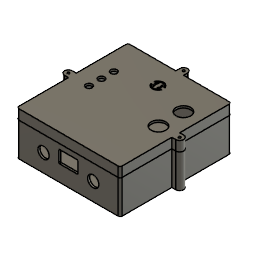
Smart_Chair_Case (Autodesk Fusion 360 design; units mm, degrees)
Autodesk Fusion 360 part; units mm, degrees
note: some values were not read from the file. Set by a fixed rule: which face or edge a step refers to.
sketch "Sketch1" plane through (200, 0, 0) normal (1, 0, 0) x (0, 0, -1)
  line L0 (113.9291, 131.1741) -> (113.9291, 10) construction
  circle A0 centre (113.9291, 70.587) radius 30
  circle A1 centre (113.9291, 70.587) radius 27.5
  circle A2 centre (113.9291, 70.587) radius 25
  circle A3 centre (113.9291, 70.587) radius 22.5
  circle A4 centre (113.9291, 70.587) radius 20
  circle A5 centre (113.9291, 70.587) radius 17.5
  circle A6 centre (113.9291, 70.587) radius 15
  circle A7 centre (113.9291, 70.587) radius 15
  circle A8 centre (113.9291, 70.587) radius 12.5
  circle A9 centre (113.9291, 70.587) radius 10
  circle A10 centre (113.9291, 70.587) radius 7.5
  circle A11 centre (113.9291, 70.587) radius 5
  circle A12 centre (113.9291, 70.587) radius 2.5
  line L1 (71.2868, 76.587) -> (156.5714, 76.587)
  line L2 (156.5714, 76.587) -> (156.5714, 64.587)
  line L3 (156.5714, 64.587) -> (71.2868, 64.587)
  line L4 (71.2868, 64.587) -> (71.2868, 76.587)
  line L5 (71.2868, 76.587) -> (156.5714, 64.587) construction
  line L6 (156.5714, 76.587) -> (71.2868, 64.587) construction
  line L7 (107.9291, 108.7596) -> (119.9291, 108.7596)
  line L8 (119.9291, 108.7596) -> (119.9291, 32.4145)
  line L9 (119.9291, 32.4145) -> (107.9291, 32.4145)
  line L10 (107.9291, 32.4145) -> (107.9291, 108.7596)
  line L11 (107.9291, 108.7596) -> (119.9291, 32.4145) construction
  line L12 (119.9291, 108.7596) -> (107.9291, 32.4145) construction
  line L13 (-90, 0) -> (90, 0)
  line L14 (90, 0) -> (90, 150)
  line L15 (-90, 125) -> (-90, 0)
  line L16 (90, 150) -> (-90, 125)
  point P0 (113.9291, 70.587)
  point P1 (113.9291, 70.587)
  dimension "d204" = 60
  dimension "d205" = 55
  dimension "d206" = 50
  dimension "d207" = 45
  dimension "d208" = 40
  dimension "d209" = 35
  dimension "d210" = 30
  dimension "d211" = 30
  dimension "d212" = 25
  dimension "d213" = 20
  dimension "d214" = 15
  dimension "d215" = 10
  dimension "d216" = 5
  dimension "d217" = 12
  dimension "d218" = 12
  constraint midpoint L0 P1
  constraint concentric A0 A1
  constraint concentric A0 A2
  constraint concentric A2 A3
  constraint concentric A1 A4
  constraint concentric A0 A5
  constraint concentric A1 A6
  constraint concentric A6 A7
  constraint concentric A0 A8
  constraint concentric A7 A9
  constraint concentric A0 A10
  constraint concentric A6 A11
  constraint concentric A3 A12
  constraint horizontal L1
  constraint perpendicular L1 L2
  constraint parallel L1 L3
  constraint parallel L2 L4
  constraint coincident L5 P1
  constraint coincident L6 P1
  constraint coincident P1 P0
  constraint horizontal L7
  constraint perpendicular L7 L8
  constraint parallel L7 L9
  constraint parallel L8 L10
  constraint coincident L11 P1
  constraint coincident L12 P1
  measures "d204" diameter of A0
  measures "d205" diameter of A1
  measures "d206" diameter of A2
  measures "d207" diameter of A3
  measures "d208" diameter of A4
  measures "d209" diameter of A5
  measures "d210" diameter of A6
  measures "d211" diameter of A7
  measures "d212" diameter of A8
  measures "d213" diameter of A9
  measures "d214" diameter of A10
  measures "d215" diameter of A11
  measures "d216" diameter of A12
  measures "d217" distance of L1.end L2.end
  measures "d218" distance of L8.end L9.end
sketch "Sketch1 (2)" plane through (0, 0, 0) normal (0, 1, 0) x (1, 0, 0) in component "Smart_Sprayer_Board_Case"
  line L0 (-77.5, 47.5) -> (77.5, 47.5)
  line L1 (77.5, 47.5) -> (77.5, -47.5)
  line L2 (77.5, -47.5) -> (-77.5, -47.5)
  line L3 (-77.5, -47.5) -> (-77.5, 47.5)
  line L4 (-77.5, 47.5) -> (77.5, -47.5) construction
  line L5 (77.5, 47.5) -> (-77.5, -47.5) construction
  line L6 (-79.25, 49.25) -> (79.25, 49.25)
  line L7 (79.25, 49.25) -> (79.25, -49.25)
  line L8 (79.25, -49.25) -> (-79.25, -49.25)
  line L9 (-79.25, -49.25) -> (-79.25, 49.25)
  line L10 (-79.25, 49.25) -> (79.25, -49.25) construction
  line L11 (79.25, 49.25) -> (-79.25, -49.25) construction
  dimension "d292" = 155
  dimension "d293" = 95
  dimension "d294" = 158.5
  dimension "d295" = 98.5
  constraint horizontal L0
  constraint perpendicular L0 L1
  constraint parallel L0 L2
  constraint parallel L1 L3
  constraint coincident L4 origin
  constraint coincident L5 origin
  constraint horizontal L6
  constraint perpendicular L6 L7
  constraint parallel L6 L8
  constraint parallel L7 L9
  constraint coincident L10 origin
  constraint coincident L11 origin
  measures "d292" distance of L1.end L2.end
  measures "d293" distance of L0.end L1.end
  measures "d294" distance of L7.end L8.end
  measures "d295" distance of L6.end L7.end
extrude "Extrude1" add sketch "Sketch1 (2)" along normal blind 43 makes body 1 in component "Smart_Sprayer_Board_Case"
sketch "Sketch2" plane through (0, 0, 0) normal (0, -1, 0) x (1, 0, 0) in component "Smart_Sprayer_Board_Case"
  line L0 (-77.5, 47.5) -> (77.5, 47.5)
  line L1 (77.5, 47.5) -> (77.5, -47.5)
  line L2 (77.5, -47.5) -> (-77.5, -47.5)
  line L3 (-77.5, -47.5) -> (-77.5, 47.5)
  line L4 (79.25, 49.25) -> (-79.25, 49.25)
  line L5 (-79.25, 49.25) -> (-79.25, -49.25)
  line L6 (-79.25, -49.25) -> (79.25, -49.25)
  line L7 (79.25, -49.25) -> (79.25, 49.25)
extrude "Extrude2" add sketch "Sketch2" along normal blind 1.75 contours L0 L1 L2 L3 | L4 L5 L6 L7 bodies 1 in component "Smart_Sprayer_Board_Case"
sketch "Sketch3" plane through (0, 0, 0) normal (0, 1, 0) x (-1, 0, 0) in component "Smart_Sprayer_Board_Case"
  line L0 (-77.5, 47.5) -> (-77.5, -47.5)
  line L1 (-77.5, -47.5) -> (77.5, -47.5)
  line L2 (77.5, -47.5) -> (77.5, 47.5)
  line L3 (77.5, 47.5) -> (-77.5, 47.5)
  line L4 (70, -41.25) -> (-70, -41.25) construction
  line L5 (-70, -41.25) -> (-70, 41.25) construction
  line L6 (-70, 41.25) -> (70, 41.25) construction
  line L7 (70, 41.25) -> (70, -41.25) construction
  line L8 (70, -41.25) -> (-70, 41.25) construction
  line L9 (-70, -41.25) -> (70, 41.25) construction
  circle A0 centre (70, -41.25) radius 5
  circle A1 centre (-70, -41.25) radius 5
  circle A2 centre (70, 41.25) radius 5
  circle A3 centre (-70, 41.25) radius 5
  dimension "d300" = 140
  dimension "d301" = 82.5
  dimension "d302" = 10
  dimension "d303" = 10
  dimension "d304" = 10
  dimension "d305" = 10
  constraint horizontal L4
  constraint perpendicular L4 L5
  constraint parallel L4 L6
  constraint parallel L5 L7
  constraint coincident L8 origin
  constraint coincident L9 origin
  constraint coincident L4.start L7.end
  constraint coincident L4.end L5.start
  constraint coincident L6.end L7.start
  constraint coincident L5.end L6.start
  measures "d300" distance of L5.end L6.end
  measures "d301" distance of L4.end L5.end
  measures "d302" diameter of A0
  measures "d303" diameter of A1
  measures "d304" diameter of A2
  measures "d305" diameter of A3
extrude "Extrude3" add sketch "Sketch3" along normal blind 3 contours A0 | A1 | A2 | A3 bodies 1 in component "Smart_Sprayer_Board_Case"
sketch "Sketch4" plane through (0, 3, 0) normal (0, 1, 0) x (-1, 0, 0) in component "Smart_Sprayer_Board_Case"
  circle A0 centre (70, -41.25) radius 5
  circle A1 centre (70, -41.25) radius 1
  dimension "d308" = 2
  constraint concentric A0 A1
  measures "d308" diameter of A1
extrude "Extrude4" cut sketch "Sketch4" against normal blind 4 contours A1 bodies 1 in component "Smart_Sprayer_Board_Case"
pattern_linear "R-Pattern1" count 2 spacing 82.5 along (0, 0, 1) count 2 spacing 140 along (1, 0, 0) of "Extrude4" in component "Smart_Sprayer_Board_Case"
sketch "Sketch5" plane through (0, 0, 47.5) normal (0, 0, -1) x (-1, 0, 0) in component "Smart_Sprayer_Board_Case"
  line L0 (-77.5, 0) -> (77.5, 0)
  line L1 (77.5, 0) -> (77.5, 43)
  line L2 (77.5, 43) -> (-77.5, 43)
  line L3 (-77.5, 43) -> (-77.5, 0)
  line L4 (0, 0) -> (0, 18) construction
  line L5 (-8, 25) -> (8, 25)
  line L6 (8, 25) -> (8, 11)
  line L7 (8, 11) -> (-8, 11)
  line L8 (-8, 11) -> (-8, 25)
  line L9 (-8, 25) -> (8, 11) construction
  line L10 (8, 25) -> (-8, 11) construction
  point P0 (0, 18)
  dimension "d315" = 18
  dimension "d316" = 16
  dimension "d317" = 14
  constraint coincident L4.start origin
  constraint perpendicular L0 L4
  constraint horizontal L5
  constraint perpendicular L5 L6
  constraint parallel L5 L7
  constraint parallel L6 L8
  constraint coincident L9 P0
  constraint coincident L10 P0
  constraint coincident P0 L4.end
  measures "d315" distance of L4.start P0
  measures "d316" distance of L6.end L7.end
  measures "d317" distance of L5.end L6.end
extrude "Extrude5" cut sketch "Sketch5" against normal blind 1.75 contours L5 L6 L7 L8 bodies 1 in component "Smart_Sprayer_Board_Case"
sketch "Sketch6" plane through (-79.25, 0, 0) normal (-1, 0, 0) x (0, 0, 1) in component "Smart_Sprayer_Board_Case"
  line L0 (49.25, -1.75) -> (49.25, 43)
  line L1 (49.25, 43) -> (-49.25, 43)
  line L2 (-49.25, 43) -> (-49.25, -1.75)
  line L3 (-49.25, -1.75) -> (49.25, -1.75)
  line L4 (0, 0) -> (0, 25) construction
  line L5 (0, 25) -> (49.25, 25) construction
  line L6 (0, 25) -> (-49.25, 25) construction
  line L7 (0, 25) -> (-21, 25) construction
  line L8 (0, 25) -> (21, 25) construction
  line L9 (-26.5, 30.5) -> (-15.5, 30.5)
  line L10 (-15.5, 30.5) -> (-15.5, 19.5)
  line L11 (-15.5, 19.5) -> (-26.5, 19.5)
  line L12 (-26.5, 19.5) -> (-26.5, 30.5)
  line L13 (-26.5, 30.5) -> (-15.5, 19.5) construction
  line L14 (-15.5, 30.5) -> (-26.5, 19.5) construction
  line L15 (15.5, 30.5) -> (26.5, 30.5)
  line L16 (26.5, 30.5) -> (26.5, 19.5)
  line L17 (26.5, 19.5) -> (15.5, 19.5)
  line L18 (15.5, 19.5) -> (15.5, 30.5)
  line L19 (15.5, 30.5) -> (26.5, 19.5) construction
  line L20 (26.5, 30.5) -> (15.5, 19.5) construction
  point P0 (-21, 25)
  point P1 (21, 25)
  dimension "d320" = 25
  dimension "d321" = 21
  dimension "d322" = 21
  dimension "d323" = 11
  dimension "d324" = 11
  dimension "d325" = 11
  dimension "d326" = 11
  constraint coincident L4.start origin
  constraint perpendicular L3 L4
  constraint coincident L0 L5.end
  constraint perpendicular L0 L5
  constraint coincident L2 L6.end
  constraint perpendicular L2 L6
  constraint perpendicular L4 L7
  constraint perpendicular L4 L8
  constraint horizontal L9
  constraint perpendicular L9 L10
  constraint parallel L9 L11
  constraint parallel L10 L12
  constraint coincident L13 P0
  constraint coincident L14 P0
  constraint coincident P0 L7.end
  constraint horizontal L15
  constraint perpendicular L15 L16
  constraint parallel L15 L17
  constraint parallel L16 L18
  constraint coincident L19 P1
  constraint coincident L20 P1
  constraint coincident P1 L8.end
  measures "d320" distance of L4.start L4.end
  measures "d321" distance of L4.end P0
  measures "d322" distance of L4.end P1
  measures "d323" distance of L10.end L11.end
  measures "d324" distance of L9.end L10.end
  measures "d325" distance of L16.end L17.end
  measures "d326" distance of L15.end L16.end
extrude "Extrude6" cut sketch "Sketch6" against normal blind 1.75 contours L9 L10 L11 L12 | L15 L16 L17 L18 bodies 1 in component "Smart_Sprayer_Board_Case"
sketch "Sketch7" plane through (0, 0, 49.25) normal (0, 0, 1) x (1, 0, 0) in component "Smart_Sprayer_Board_Case"
  line L0 (-8, 11) -> (-8, 25)
  line L1 (-8, 25) -> (8, 25)
  line L2 (8, 25) -> (8, 11)
  line L3 (8, 11) -> (-8, 11)
  line L4 (79.25, -1.75) -> (79.25, 43)
  line L5 (79.25, 43) -> (-79.25, 43)
  line L6 (-79.25, 43) -> (-79.25, -1.75)
  line L7 (-79.25, -1.75) -> (79.25, -1.75)
  line L8 (-8, 18) -> (-79.25, 18) construction
  line L9 (-8, 18) -> (-15, 18) construction
  circle A0 centre (-15, 18) radius 3.5
  dimension "d329" = 7
  dimension "d330" = 7
  constraint midpoint L0 L8.start
  constraint coincident L6 L8.end
  constraint perpendicular L6 L8
  constraint perpendicular L0 L9
  constraint coincident L9.end A0.centre
  measures "d329" distance of L8.start L9.end
  measures "d330" diameter of A0
extrude "Extrude7" cut sketch "Sketch7" against normal blind 1.75 contours A0 bodies 1 in component "Smart_Sprayer_Board_Case"
sketch "Sketch8" plane through (79.25, 0, 0) normal (1, 0, 0) x (0, 0, -1) in component "Smart_Sprayer_Board_Case"
  line L0 (49.25, -1.75) -> (49.25, 43)
  line L1 (49.25, 43) -> (-49.25, 43)
  line L2 (-49.25, 43) -> (-49.25, -1.75)
  line L3 (-49.25, -1.75) -> (49.25, -1.75)
  line L4 (16.5, 29.5) -> (33.5, 29.5)
  line L5 (33.5, 29.5) -> (33.5, 20.5)
  line L6 (33.5, 20.5) -> (16.5, 20.5)
  line L7 (16.5, 20.5) -> (16.5, 29.5)
  line L8 (16.5, 29.5) -> (33.5, 20.5) construction
  line L9 (33.5, 29.5) -> (16.5, 20.5) construction
  point P0 (25, 25)
  dimension "d333" = 17
  dimension "d334" = 9
  constraint horizontal L4
  constraint perpendicular L4 L5
  constraint parallel L4 L6
  constraint parallel L5 L7
  constraint coincident L8 P0
  constraint coincident L9 P0
  measures "d333" distance of L5.end L6.end
  measures "d334" distance of L4.end L5.end
extrude "Extrude8" cut sketch "Sketch8" against normal blind 1.75 contours L4 L5 L6 L7 bodies 1 in component "Smart_Sprayer_Board_Case"
sketch "Sketch9" plane through (0, -1.75, 0) normal (0, -1, 0) x (1, 0, 0) in component "Smart_Sprayer_Board_Case"
  line L0 (79.25, -49.25) -> (79.25, 49.25)
  line L1 (79.25, 49.25) -> (-79.25, 49.25)
  line L2 (-79.25, 49.25) -> (-79.25, -49.25)
  line L3 (-79.25, -49.25) -> (79.25, -49.25)
  line L4 (79.25, -49.25) -> (-79.25, -49.25)
  line L5 (-79.25, -49.25) -> (-79.25, -74.45)
  line L6 (-79.25, -74.45) -> (79.25, -74.45)
  line L7 (79.25, -74.45) -> (79.25, -49.25)
  dimension "d337" = 25.2
  constraint horizontal L4
  constraint vertical L5
  constraint horizontal L6
  constraint vertical L7
  constraint coincident L0.start L3.end
  measures "d337" distance of L0.start L6.end
extrude "Extrude9" add sketch "Sketch9" against normal blind 7 contours L3 L4 L5 L6 L7 bodies 1 in component "Smart_Sprayer_Board_Case"
sketch "Sketch10" plane through (0, 5.25, 0) normal (0, 1, 0) x (-1, 0, 0) in component "Smart_Sprayer_Board_Case"
  line L0 (-79.25, -49.25) -> (-79.25, -74.45)
  line L1 (-79.25, -74.45) -> (79.25, -74.45)
  line L2 (79.25, -74.45) -> (79.25, -49.25)
  line L3 (79.25, -49.25) -> (-79.25, -49.25)
  line L4 (79.25, -74.45) -> (-79.25, -49.25) construction
  circle A0 centre (0, -61.85) radius 2.5
  line L5 (0, -61.85) -> (-79.25, -61.85) construction
  line L6 (0, -61.85) -> (79.25, -61.85) construction
  circle A1 centre (39.625, -61.85) radius 2.5
  circle A2 centre (-39.625, -61.85) radius 2.5
  dimension "d340" = 5
  dimension "d341" = 5
  dimension "d342" = 5
  constraint coincident L1.end L2.start
  constraint coincident L0.start L3.end
  constraint midpoint L4 A0.centre
  constraint coincident A0.centre L5.start
  constraint midpoint L0 L5.end
  constraint midpoint L2 L6.end
  constraint midpoint L6 A1.centre
  constraint midpoint L5 A2.centre
  measures "d340" diameter of A0
  measures "d341" diameter of A1
  measures "d342" diameter of A2
extrude "Extrude10" cut sketch "Sketch10" against normal blind 7 contours A0 | A1 | A2 bodies 1 in component "Smart_Sprayer_Board_Case"
chamfer "Chamfer1" distance 20 angle 45 2 edges at (79.25, 1.75, -74.45) (-79.25, 1.75, -74.45) on bodies 1 in component "Smart_Sprayer_Board_Case"
fillet "Fillet1" radius 1.75 14 edges at (-79.25, 24.125, -49.25) (-79.25, 5.25, -51.85) (-69.25, 5.25, -64.45) (-79.25, 1.75, -54.45) (-59.25, 1.75, -74.45) (0, 5.25, -74.45) (69.25, 5.25, -64.45) (59.25, 1.75, -74.45) (79.25, 1.75, -54.45) (79.25, 5.25, -51.85) (0, 5.25, -49.25) (79.25, 24.125, -49.25) (79.25, 20.625, 49.25) (-79.25, 20.625, 49.25) on bodies 1 in component "Smart_Sprayer_Board_Case"
fillet "Fillet2" radius 0.75 20 edges at (-8, 25, 48.375) (-8, 11, 48.375) (8, 11, 48.375) (8, 25, 48.375) (-78.375, 30.5, 15.5) (-78.375, 30.5, -26.5) (-78.375, 30.5, -15.5) (-78.375, 30.5, 26.5) (-78.375, 19.5, 26.5) (-78.375, 19.5, 15.5) (-78.375, 19.5, -26.5) (-78.375, 19.5, -15.5) (78.375, 29.5, -33.5) (78.375, 29.5, -16.5) (78.375, 20.5, -16.5) (78.375, 20.5, -33.5) (77.5, 21.5, -47.5) (77.5, 21.5, 47.5) (-77.5, 21.5, 47.5) (-77.5, 21.5, -47.5) on bodies 1 in component "Smart_Sprayer_Board_Case"
sketch "Sketch1 (3)" plane through (0, 0, 0) normal (0, 1, 0) x (1, 0, 0) in component "Smart_Chair_Board_Case_Top"
  line L0 (-44, 47.5) -> (44, 47.5)
  line L1 (44, 47.5) -> (44, -47.5)
  line L2 (44, -47.5) -> (-44, -47.5)
  line L3 (-44, -47.5) -> (-44, 47.5)
  line L4 (-44, 47.5) -> (44, -47.5) construction
  line L5 (44, 47.5) -> (-44, -47.5) construction
  line L6 (-45.75, 49.25) -> (45.75, 49.25)
  line L7 (45.75, 49.25) -> (45.75, -49.25)
  line L8 (45.75, -49.25) -> (-45.75, -49.25)
  line L9 (-45.75, -49.25) -> (-45.75, 49.25)
  line L10 (-45.75, 49.25) -> (45.75, -49.25) construction
  line L11 (45.75, 49.25) -> (-45.75, -49.25) construction
  dimension "d350" = 88
  dimension "d351" = 95
  dimension "d352" = 91.5
  dimension "d353" = 98.5
  constraint horizontal L0
  constraint perpendicular L0 L1
  constraint parallel L0 L2
  constraint parallel L1 L3
  constraint coincident L4 origin
  constraint coincident L5 origin
  constraint horizontal L6
  constraint perpendicular L6 L7
  constraint parallel L6 L8
  constraint parallel L7 L9
  constraint coincident L10 origin
  constraint coincident L11 origin
  measures "d350" distance of L1.end L2.end
  measures "d351" distance of L0.end L1.end
  measures "d352" distance of L7.end L8.end
  measures "d353" distance of L6.end L7.end
extrude "Extrude1'" add sketch "Sketch1 (3)" along normal blind 28 separate body makes body 2 in component "Smart_Chair_Board_Case_Top"
sketch "Sketch2 (2)" plane through (0, 0, 0) normal (0, -1, 0) x (1, 0, 0) in component "Smart_Chair_Board_Case_Top"
  line L0 (-44, 47.5) -> (44, 47.5)
  line L1 (44, 47.5) -> (44, -47.5)
  line L2 (44, -47.5) -> (-44, -47.5)
  line L3 (-44, -47.5) -> (-44, 47.5)
  line L4 (45.75, 49.25) -> (-45.75, 49.25)
  line L5 (-45.75, 49.25) -> (-45.75, -49.25)
  line L6 (-45.75, -49.25) -> (45.75, -49.25)
  line L7 (45.75, -49.25) -> (45.75, 49.25)
extrude "Extrude2'" add sketch "Sketch2 (2)" along normal blind 1.75 contours L0 L1 L2 L3 | L4 L5 L6 L7 bodies 2 in component "Smart_Chair_Board_Case_Top"
sketch "Sketch3 (2)" plane through (0, 0, 0) normal (0, 1, 0) x (-1, 0, 0) in component "Smart_Chair_Board_Case_Top"
  line L0 (-44, 47.5) -> (-44, -47.5)
  line L1 (-44, -47.5) -> (44, -47.5)
  line L2 (44, -47.5) -> (44, 47.5)
  line L3 (44, 47.5) -> (-44, 47.5)
  line L4 (39.5, -39.5) -> (-39.5, -39.5) construction
  line L5 (-39.5, -39.5) -> (-39.5, 39.5) construction
  line L6 (-39.5, 39.5) -> (39.5, 39.5) construction
  line L7 (39.5, 39.5) -> (39.5, -39.5) construction
  line L8 (39.5, -39.5) -> (-39.5, 39.5) construction
  line L9 (-39.5, -39.5) -> (39.5, 39.5) construction
  circle A0 centre (39.5, -39.5) radius 3.5
  circle A1 centre (-39.5, -39.5) radius 3.5
  circle A2 centre (39.5, 39.5) radius 3.5
  circle A3 centre (-39.5, 39.5) radius 3.5
  circle A4 centre (39.5, -39.5) radius 1
  circle A5 centre (-39.5, -39.5) radius 1
  circle A6 centre (39.5, 39.5) radius 1
  circle A7 centre (-39.5, 39.5) radius 1
  dimension "d358" = 79
  dimension "d359" = 79
  dimension "d360" = 7
  dimension "d361" = 7
  dimension "d362" = 7
  dimension "d363" = 7
  dimension "d364" = 2
  dimension "d365" = 2
  dimension "d366" = 2
  dimension "d367" = 2
  constraint horizontal L4
  constraint perpendicular L4 L5
  constraint parallel L4 L6
  constraint parallel L5 L7
  constraint coincident L8 origin
  constraint coincident L9 origin
  constraint coincident L4.start L7.end
  constraint coincident L4.end L5.start
  constraint coincident L6.end L7.start
  constraint coincident L5.end L6.start
  constraint concentric A0 A4
  constraint concentric A1 A5
  constraint concentric A2 A6
  constraint concentric A3 A7
  measures "d358" distance of L5.end L6.end
  measures "d359" distance of L4.end L5.end
  measures "d360" diameter of A0
  measures "d361" diameter of A1
  measures "d362" diameter of A2
  measures "d363" diameter of A3
  measures "d364" diameter of A4
  measures "d365" diameter of A5
  measures "d366" diameter of A6
  measures "d367" diameter of A7
extrude "Extrude3'" add sketch "Sketch3 (2)" along normal blind 3 contours A0 | A1 | A2 | A3 bodies 2 in component "Smart_Chair_Board_Case_Top"
sketch "Sketch4 (2)" plane through (0, 0, 49.25) normal (0, 0, 1) x (1, 0, 0) in component "Smart_Chair_Board_Case_Top"
  line L0 (45.75, -1.75) -> (45.75, 28)
  line L1 (45.75, 28) -> (-45.75, 28)
  line L2 (-45.75, 28) -> (-45.75, -1.75)
  line L3 (-45.75, -1.75) -> (45.75, -1.75)
  line L4 (0, 0) -> (0, 18) construction
  line L5 (-8.5, 23.5) -> (8.5, 23.5)
  line L6 (8.5, 23.5) -> (8.5, 12.5)
  line L7 (8.5, 12.5) -> (-8.5, 12.5)
  line L8 (-8.5, 12.5) -> (-8.5, 23.5)
  line L9 (-8.5, 23.5) -> (8.5, 12.5) construction
  line L10 (8.5, 23.5) -> (-8.5, 12.5) construction
  point P0 (0, 18)
  dimension "d370" = 18
  dimension "d371" = 17
  dimension "d372" = 11
  constraint coincident L4.start origin
  constraint vertical L4
  constraint horizontal L5
  constraint perpendicular L5 L6
  constraint parallel L5 L7
  constraint parallel L6 L8
  constraint coincident L9 P0
  constraint coincident L10 P0
  constraint coincident P0 L4.end
  measures "d370" distance of L4.start P0
  measures "d371" distance of L6.end L7.end
  measures "d372" distance of L5.end L6.end
extrude "Extrude4'" cut sketch "Sketch4 (2)" against normal blind 1.75 contours L5 L6 L7 L8 bodies 2 in component "Smart_Chair_Board_Case_Top"
sketch "Sketch5 (2)" plane through (0, 0, 47.5) normal (0, 0, -1) x (-1, 0, 0) in component "Smart_Chair_Board_Case_Top"
  line L0 (-8.5, 12.5) -> (-8.5, 23.5)
  line L1 (-8.5, 23.5) -> (8.5, 23.5)
  line L2 (8.5, 23.5) -> (8.5, 12.5)
  line L3 (8.5, 12.5) -> (-8.5, 12.5)
  line L4 (-44, 0) -> (44, 0)
  line L5 (44, 0) -> (44, 28)
  line L6 (44, 28) -> (-44, 28)
  line L7 (-44, 28) -> (-44, 0)
  line L8 (-44, 28) -> (0, 0) construction
  circle A0 centre (-22, 14) radius 5
  line L9 (0, 0) -> (44, 28) construction
  circle A1 centre (22, 14) radius 5
  dimension "d375" = 10
  dimension "d376" = 10
  constraint coincident L6.end L7.start
  constraint coincident L8.end L9.start
  constraint midpoint L8 A0.centre
  constraint coincident L5.end L6.start
  constraint midpoint L9 A1.centre
  measures "d375" diameter of A0
  measures "d376" diameter of A1
extrude "Extrude5'" cut sketch "Sketch5 (2)" against normal blind 1.75 contours A0 | A1 bodies 2 in component "Smart_Chair_Board_Case_Top"
sketch "Sketch6 (2)" plane through (0, 0, 47.5) normal (0, 0, -1) x (-1, 0, 0) in component "Smart_Chair_Board_Case_Top"
  circle A0 centre (-22, 14) radius 5
  circle A1 centre (22, 14) radius 5
  line L0 (-8.5, 12.5) -> (-8.5, 23.5)
  line L1 (-8.5, 23.5) -> (8.5, 23.5)
  line L2 (8.5, 23.5) -> (8.5, 12.5)
  line L3 (8.5, 12.5) -> (-8.5, 12.5)
  line L4 (-44, 0) -> (44, 0)
  line L5 (44, 0) -> (44, 28)
  line L6 (44, 28) -> (-44, 28)
  line L7 (-44, 28) -> (-44, 0)
extrude "Extrude6'" cut sketch "Sketch6 (2)" along normal blind 96.75 contours A0 bodies 2 in component "Smart_Chair_Board_Case_Top"
sketch "Sketch7 (2)" plane through (45.75, 0, 0) normal (1, 0, 0) x (0, 0, -1) in component "Smart_Chair_Board_Case_Top"
  line L0 (49.25, -1.75) -> (49.25, 28)
  line L1 (49.25, 28) -> (-49.25, 28)
  line L2 (-49.25, 28) -> (-49.25, -1.75)
  line L3 (-49.25, -1.75) -> (49.25, -1.75)
sketch "Sketch8 (2)" plane through (-45.75, 0, 0) normal (-1, 0, 0) x (0, 0, 1) in component "Smart_Chair_Board_Case_Top"
  line L0 (49.25, -1.75) -> (49.25, 28)
  line L1 (49.25, 28) -> (-49.25, 28)
  line L2 (-49.25, 28) -> (-49.25, -1.75)
  line L3 (-49.25, -1.75) -> (49.25, -1.75)
  line L4 (42.6586, 15.825) -> (28.4086, 15.825)
  line L5 (28.4086, 15.825) -> (28.4086, 24.325)
  line L6 (28.4086, 24.325) -> (42.6586, 24.325)
  line L7 (42.6586, 24.325) -> (42.6586, 15.825)
  dimension "d381" = 14.25
  dimension "d382" = 8.5
  constraint horizontal L4
  constraint vertical L5
  constraint horizontal L6
  constraint vertical L7
  measures "d381" distance of L4.start L4.end
  measures "d382" distance of L4.start L6.end
extrude "Extrude7'" cut sketch "Sketch8 (2)" against normal blind 1.75 contours L4 L5 L6 L7 bodies 2 in component "Smart_Chair_Board_Case_Top"
sketch "Sketch9 (2)" plane through (-45.75, 0, 0) normal (-1, 0, 0) x (0, 0, 1) in component "Smart_Chair_Board_Case_Top"
  line L0 (28.4086, 15.825) -> (28.4086, 24.325)
  line L1 (28.4086, 24.325) -> (42.6586, 24.325)
  line L2 (42.6586, 24.325) -> (42.6586, 15.825)
  line L3 (42.6586, 15.825) -> (28.4086, 15.825)
  line L4 (49.25, -1.75) -> (49.25, 28)
  line L5 (49.25, 28) -> (-49.25, 28)
  line L6 (-49.25, 28) -> (-49.25, -1.75)
  line L7 (-49.25, -1.75) -> (49.25, -1.75)
  circle A0 centre (14.4489, 20.075) radius 4.1
  dimension "d385" = 8.2
  measures "d385" diameter of A0
extrude "Extrude8'" cut sketch "Sketch9 (2)" against normal blind 1.75 contours A0 bodies 2 in component "Smart_Chair_Board_Case_Top"
fillet "Fillet1'" radius 1.75 8 edges at (-45.75, 13.125, 49.25) (-45.75, 13.125, -49.25) (45.75, 13.125, -49.25) (45.75, 13.125, 49.25) (-44, 14, -47.5) (44, 14, -47.5) (44, 14, 47.5) (-44, 14, 47.5) on bodies 2 in component "Smart_Chair_Board_Case_Top"
fillet "Fillet2'" radius 0.75 4 edges at (-8.5, 23.5, 48.375) (-8.5, 12.5, 48.375) (8.5, 12.5, 48.375) (8.5, 23.5, 48.375) on bodies 2 in component "Smart_Chair_Board_Case_Top"
sketch "Sketch10 (2)" plane through (0, 28, 0) normal (0, 1, 0) x (-1, 0, 0) in component "Smart_Chair_Board_Case_Top"
  arc A0 (-44, 49.25) -> (-45.75, 47.5) centre (-44, 47.5) ccw
  line L0 (-45.75, 47.5) -> (-45.75, -47.5)
  arc A1 (-45.75, -47.5) -> (-44, -49.25) centre (-44, -47.5) ccw
  line L1 (-44, -49.25) -> (44, -49.25)
  arc A2 (44, -49.25) -> (45.75, -47.5) centre (44, -47.5) ccw
  line L2 (45.75, -47.5) -> (45.75, 47.5)
  arc A3 (45.75, 47.5) -> (44, 49.25) centre (44, 47.5) ccw
  line L3 (44, 49.25) -> (-44, 49.25)
  line L4 (-42.25, 47.5) -> (42.25, 47.5)
  arc A4 (44, 45.75) -> (42.25, 47.5) centre (42.25, 45.75) ccw
  line L5 (44, 45.75) -> (44, -45.75)
  arc A5 (42.25, -47.5) -> (44, -45.75) centre (42.25, -45.75) ccw
  line L6 (42.25, -47.5) -> (-42.25, -47.5)
  arc A6 (-44, -45.75) -> (-42.25, -47.5) centre (-42.25, -45.75) ccw
  line L7 (-44, -45.75) -> (-44, 45.75)
  arc A7 (-42.25, 47.5) -> (-44, 45.75) centre (-42.25, 45.75) ccw
  line L8 (52.75, -3.5) -> (38.75, -3.5)
  line L9 (38.75, -3.5) -> (38.75, 3.5)
  line L10 (38.75, 3.5) -> (52.75, 3.5)
  line L11 (52.75, 3.5) -> (52.75, -3.5)
  line L12 (52.75, -3.5) -> (38.75, 3.5) construction
  line L13 (38.75, -3.5) -> (52.75, 3.5) construction
  line L14 (3.5, -56.25) -> (-3.5, -56.25)
  line L15 (-3.5, -56.25) -> (-3.5, -42.25)
  line L16 (-3.5, -42.25) -> (3.5, -42.25)
  line L17 (3.5, -42.25) -> (3.5, -56.25)
  line L18 (3.5, -56.25) -> (-3.5, -42.25) construction
  line L19 (-3.5, -56.25) -> (3.5, -42.25) construction
  line L20 (-38.75, -3.5) -> (-52.75, -3.5)
  line L21 (-52.75, -3.5) -> (-52.75, 3.5)
  line L22 (-52.75, 3.5) -> (-38.75, 3.5)
  line L23 (-38.75, 3.5) -> (-38.75, -3.5)
  line L24 (-38.75, -3.5) -> (-52.75, 3.5) construction
  line L25 (-52.75, -3.5) -> (-38.75, 3.5) construction
  point P0 (45.75, 0)
  point P1 (0, -49.25)
  point P2 (-45.75, 0)
  dimension "d392" = 14
  dimension "d393" = 7
  dimension "d394" = 7
  dimension "d395" = 14
  dimension "d396" = 14
  dimension "d397" = 7
  constraint horizontal L8
  constraint perpendicular L8 L9
  constraint parallel L8 L10
  constraint parallel L9 L11
  constraint coincident L12 P0
  constraint coincident L13 P0
  constraint midpoint L2 P0
  constraint horizontal L14
  constraint perpendicular L14 L15
  constraint parallel L14 L16
  constraint parallel L15 L17
  constraint coincident L18 P1
  constraint coincident L19 P1
  constraint midpoint L1 P1
  constraint horizontal L20
  constraint perpendicular L20 L21
  constraint parallel L20 L22
  constraint parallel L21 L23
  constraint coincident L24 P2
  constraint coincident L25 P2
  constraint midpoint L0 P2
  measures "d392" distance of L9.end L10.end
  measures "d393" distance of L8.end L9.end
  measures "d394" distance of L15.end L16.end
  measures "d395" distance of L14.end L15.end
  measures "d396" distance of L21.end L22.end
  measures "d397" distance of L20.end L21.end
extrude "Extrude9'" add sketch "Sketch10 (2)" against normal blind 29.75 contours L0 L20 L21 L22 | L2 L8 L10 L11 | L1 L14 L15 L17 bodies 2 in component "Smart_Chair_Board_Case_Top"
fillet "Fillet3" radius 3.5 6 edges at (-52.75, 13.125, 3.5) (-52.75, 13.125, -3.5) (-3.5, 13.125, -56.25) (3.5, 13.125, -56.25) (52.75, 13.125, -3.5) (52.75, 13.125, 3.5) on bodies 2 in component "Smart_Chair_Board_Case_Top"
sketch "Sketch11" plane through (0, 28, 0) normal (0, 1, 0) x (-1, 0, 0) in component "Smart_Chair_Board_Case_Top"
  arc A0 (-49.25, 3.5) -> (-49.25, -3.5) centre (-49.25, 0) ccw
  line L0 (-49.25, -3.5) -> (-45.75, -3.5)
  line L1 (-45.75, -3.5) -> (-45.75, -47.5)
  arc A1 (-45.75, -47.5) -> (-44, -49.25) centre (-44, -47.5) ccw
  line L2 (-44, -49.25) -> (-3.5, -49.25)
  line L3 (-3.5, -49.25) -> (-3.5, -52.75)
  arc A2 (-3.5, -52.75) -> (3.5, -52.75) centre (0, -52.75) ccw
  line L4 (3.5, -52.75) -> (3.5, -49.25)
  line L5 (3.5, -49.25) -> (44, -49.25)
  arc A3 (44, -49.25) -> (45.75, -47.5) centre (44, -47.5) ccw
  line L6 (45.75, -47.5) -> (45.75, -3.5)
  line L7 (45.75, -3.5) -> (49.25, -3.5)
  arc A4 (49.25, -3.5) -> (49.25, 3.5) centre (49.25, 0) ccw
  line L8 (49.25, 3.5) -> (45.75, 3.5)
  line L9 (45.75, 3.5) -> (45.75, 47.5)
  arc A5 (45.75, 47.5) -> (44, 49.25) centre (44, 47.5) ccw
  line L10 (44, 49.25) -> (-44, 49.25)
  arc A6 (-44, 49.25) -> (-45.75, 47.5) centre (-44, 47.5) ccw
  line L11 (-45.75, 47.5) -> (-45.75, 3.5)
  line L12 (-45.75, 3.5) -> (-49.25, 3.5)
  line L13 (-42.25, 47.5) -> (42.25, 47.5)
  arc A7 (44, 45.75) -> (42.25, 47.5) centre (42.25, 45.75) ccw
  line L14 (44, 45.75) -> (44, -45.75)
  arc A8 (42.25, -47.5) -> (44, -45.75) centre (42.25, -45.75) ccw
  line L15 (42.25, -47.5) -> (-42.25, -47.5)
  arc A9 (-44, -45.75) -> (-42.25, -47.5) centre (-42.25, -45.75) ccw
  line L16 (-44, -45.75) -> (-44, 45.75)
  arc A10 (-42.25, 47.5) -> (-44, 45.75) centre (-42.25, 45.75) ccw
  circle A11 centre (49.25, 0) radius 1
  circle A12 centre (-49.25, 0) radius 1
  circle A13 centre (0, -52.75) radius 1
  dimension "d402" = 2
  dimension "d403" = 2
  dimension "d404" = 2
  constraint concentric A4 A11
  constraint concentric A0 A12
  constraint concentric A2 A13
  measures "d402" diameter of A11
  measures "d403" diameter of A12
  measures "d404" diameter of A13
extrude "Extrude10'" cut sketch "Sketch11" against normal blind 15 contours A11 | A12 | A13 bodies 2 in component "Smart_Chair_Board_Case_Top"
sketch "Sketch1 (4)" plane through (0, 28, 0) normal (0, 1, 0) x (-1, 0, 0) in component "Smart_Chair_Board_Case_Top_Cover"
  circle A0 centre (-49.25, 0) radius 1
  circle A1 centre (0, -52.75) radius 1
  circle A2 centre (49.25, 0) radius 1
  arc A3 (-49.25, 3.5) -> (-49.25, -3.5) centre (-49.25, 0) ccw
  line L0 (-49.25, -3.5) -> (-45.75, -3.5)
  line L1 (-45.75, -3.5) -> (-45.75, -47.5)
  arc A4 (-45.75, -47.5) -> (-44, -49.25) centre (-44, -47.5) ccw
  line L2 (-44, -49.25) -> (-3.5, -49.25)
  line L3 (-3.5, -49.25) -> (-3.5, -52.75)
  arc A5 (-3.5, -52.75) -> (3.5, -52.75) centre (0, -52.75) ccw
  line L4 (3.5, -52.75) -> (3.5, -49.25)
  line L5 (3.5, -49.25) -> (44, -49.25)
  arc A6 (44, -49.25) -> (45.75, -47.5) centre (44, -47.5) ccw
  line L6 (45.75, -47.5) -> (45.75, -3.5)
  line L7 (45.75, -3.5) -> (49.25, -3.5)
  arc A7 (49.25, -3.5) -> (49.25, 3.5) centre (49.25, 0) ccw
  line L8 (49.25, 3.5) -> (45.75, 3.5)
  line L9 (45.75, 3.5) -> (45.75, 47.5)
  arc A8 (45.75, 47.5) -> (44, 49.25) centre (44, 47.5) ccw
  line L10 (44, 49.25) -> (-44, 49.25)
  arc A9 (-44, 49.25) -> (-45.75, 47.5) centre (-44, 47.5) ccw
  line L11 (-45.75, 47.5) -> (-45.75, 3.5)
  line L12 (-45.75, 3.5) -> (-49.25, 3.5)
  line L13 (-42.25, 47.5) -> (42.25, 47.5)
  arc A10 (44, 45.75) -> (42.25, 47.5) centre (42.25, 45.75) ccw
  line L14 (44, 45.75) -> (44, -45.75)
  arc A11 (42.25, -47.5) -> (44, -45.75) centre (42.25, -45.75) ccw
  line L15 (42.25, -47.5) -> (-42.25, -47.5)
  arc A12 (-44, -45.75) -> (-42.25, -47.5) centre (-42.25, -45.75) ccw
  line L16 (-44, -45.75) -> (-44, 45.75)
  arc A13 (-42.25, 47.5) -> (-44, 45.75) centre (-42.25, 45.75) ccw
extrude "Extrude1''" add sketch "Sketch1 (4)" along normal blind 7 separate body makes body 3 in component "Smart_Chair_Board_Case_Top_Cover"
sketch "Sketch2 (3)" plane through (0, 35, 0) normal (0, 1, 0) x (-1, 0, 0) in component "Smart_Chair_Board_Case_Top_Cover"
  arc A0 (44, 45.75) -> (42.25, 47.5) centre (42.25, 45.75) ccw
  line L0 (44, 45.75) -> (44, -45.75)
  arc A1 (42.25, -47.5) -> (44, -45.75) centre (42.25, -45.75) ccw
  line L1 (42.25, -47.5) -> (-42.25, -47.5)
  arc A2 (-44, -45.75) -> (-42.25, -47.5) centre (-42.25, -45.75) ccw
  line L2 (-44, -45.75) -> (-44, 45.75)
  arc A3 (-42.25, 47.5) -> (-44, 45.75) centre (-42.25, 45.75) ccw
  line L3 (-42.25, 47.5) -> (42.25, 47.5)
  circle A4 centre (0, -52.75) radius 1
  circle A5 centre (49.25, 0) radius 1
  circle A6 centre (-49.25, 0) radius 1
  line L4 (-45.75, 3.5) -> (-49.25, 3.5)
  arc A7 (-49.25, 3.5) -> (-49.25, -3.5) centre (-49.25, 0) ccw
  line L5 (-49.25, -3.5) -> (-45.75, -3.5)
  line L6 (-45.75, -3.5) -> (-45.75, -47.5)
  arc A8 (-45.75, -47.5) -> (-44, -49.25) centre (-44, -47.5) ccw
  line L7 (-44, -49.25) -> (-3.5, -49.25)
  line L8 (-3.5, -49.25) -> (-3.5, -52.75)
  arc A9 (-3.5, -52.75) -> (3.5, -52.75) centre (0, -52.75) ccw
  line L9 (3.5, -52.75) -> (3.5, -49.25)
  line L10 (3.5, -49.25) -> (44, -49.25)
  arc A10 (44, -49.25) -> (45.75, -47.5) centre (44, -47.5) ccw
  line L11 (45.75, -47.5) -> (45.75, -3.5)
  line L12 (45.75, -3.5) -> (49.25, -3.5)
  arc A11 (49.25, -3.5) -> (49.25, 3.5) centre (49.25, 0) ccw
  line L13 (49.25, 3.5) -> (45.75, 3.5)
  line L14 (45.75, 3.5) -> (45.75, 47.5)
  arc A12 (45.75, 47.5) -> (44, 49.25) centre (44, 47.5) ccw
  line L15 (44, 49.25) -> (-44, 49.25)
  arc A13 (-44, 49.25) -> (-45.75, 47.5) centre (-44, 47.5) ccw
  line L16 (-45.75, 47.5) -> (-45.75, 3.5)
extrude "Extrude2''" add sketch "Sketch2 (3)" along normal blind 1.75 contours A0 L0 A1 L1 A2 L2 A3 L3 | L4 A7 L5 L6 A8 L7 L8 A9 L9 L10 A10 L11 L12 A11 L13 L14 A12 L15 A13 L16 bodies 3 in component "Smart_Chair_Board_Case_Top_Cover"
sketch "Sketch3 (3)" plane through (0, 36.75, 0) normal (0, 1, 0) x (-1, 0, 0) in component "Smart_Chair_Board_Case_Top_Cover"
  circle A0 centre (-49.25, 0) radius 1
  circle A1 centre (0, -52.75) radius 1
  circle A2 centre (49.25, 0) radius 1
  line L0 (-45.75, 47.5) -> (-45.75, 3.5)
  line L1 (-45.75, 3.5) -> (-49.25, 3.5)
  arc A3 (-49.25, 3.5) -> (-49.25, -3.5) centre (-49.25, 0) ccw
  line L2 (-49.25, -3.5) -> (-45.75, -3.5)
  line L3 (-45.75, -3.5) -> (-45.75, -47.5)
  arc A4 (-45.75, -47.5) -> (-44, -49.25) centre (-44, -47.5) ccw
  line L4 (-44, -49.25) -> (-3.5, -49.25)
  line L5 (-3.5, -49.25) -> (-3.5, -52.75)
  arc A5 (-3.5, -52.75) -> (3.5, -52.75) centre (0, -52.75) ccw
  line L6 (3.5, -52.75) -> (3.5, -49.25)
  line L7 (3.5, -49.25) -> (44, -49.25)
  arc A6 (44, -49.25) -> (45.75, -47.5) centre (44, -47.5) ccw
  line L8 (45.75, -47.5) -> (45.75, -3.5)
  line L9 (45.75, -3.5) -> (49.25, -3.5)
  arc A7 (49.25, -3.5) -> (49.25, 3.5) centre (49.25, 0) ccw
  line L10 (49.25, 3.5) -> (45.75, 3.5)
  line L11 (45.75, 3.5) -> (45.75, 47.5)
  arc A8 (45.75, 47.5) -> (44, 49.25) centre (44, 47.5) ccw
  line L12 (44, 49.25) -> (-44, 49.25)
  arc A9 (-44, 49.25) -> (-45.75, 47.5) centre (-44, 47.5) ccw
  line L13 (45.75, -49.25) -> (30.25, -49.25) construction
  line L14 (30.25, -49.25) -> (30.25, -21.25) construction
  line L15 (30.25, -21.25) -> (45.75, -21.25) construction
  line L16 (45.75, -21.25) -> (45.75, -49.25) construction
  circle A10 centre (30.25, -21.25) radius 2.8
  dimension "d411" = 15.5
  dimension "d412" = 28
  dimension "d413" = 5.6
  constraint horizontal L13
  constraint vertical L14
  constraint horizontal L15
  constraint vertical L16
  constraint coincident L14.end L15.start
  measures "d411" distance of L13.start L13.end
  measures "d412" distance of L13.start L15.end
  measures "d413" diameter of A10
extrude "Extrude3''" cut sketch "Sketch3 (3)" against normal blind 8.75 contours A10 bodies 3 in component "Smart_Chair_Board_Case_Top_Cover"
pattern_linear "R-Pattern1'" count 1 spacing 0 along (-1, 0, 0) count 3 spacing 11 along (0, 0, 1) of "Extrude3''" in component "Smart_Chair_Board_Case_Top_Cover"
sketch "Sketch4 (3)" plane through (0, 36.75, 0) normal (0, 1, 0) x (-1, 0, 0) in component "Smart_Chair_Board_Case_Top_Cover"
  circle A0 centre (30.25, 0.75) radius 2.8
  circle A1 centre (30.25, -10.25) radius 2.8
  circle A2 centre (30.25, -21.25) radius 2.8
  circle A3 centre (-49.25, 0) radius 1
  circle A4 centre (0, -52.75) radius 1
  circle A5 centre (49.25, 0) radius 1
  line L0 (-45.75, 47.5) -> (-45.75, 3.5)
  line L1 (-45.75, 3.5) -> (-49.25, 3.5)
  arc A6 (-49.25, 3.5) -> (-49.25, -3.5) centre (-49.25, 0) ccw
  line L2 (-49.25, -3.5) -> (-45.75, -3.5)
  line L3 (-45.75, -3.5) -> (-45.75, -47.5)
  arc A7 (-45.75, -47.5) -> (-44, -49.25) centre (-44, -47.5) ccw
  line L4 (-44, -49.25) -> (-3.5, -49.25)
  line L5 (-3.5, -49.25) -> (-3.5, -52.75)
  arc A8 (-3.5, -52.75) -> (3.5, -52.75) centre (0, -52.75) ccw
  line L6 (3.5, -52.75) -> (3.5, -49.25)
  line L7 (3.5, -49.25) -> (44, -49.25)
  arc A9 (44, -49.25) -> (45.75, -47.5) centre (44, -47.5) ccw
  line L8 (45.75, -47.5) -> (45.75, -3.5)
  line L9 (45.75, -3.5) -> (49.25, -3.5)
  arc A10 (49.25, -3.5) -> (49.25, 3.5) centre (49.25, 0) ccw
  line L10 (49.25, 3.5) -> (45.75, 3.5)
  line L11 (45.75, 3.5) -> (45.75, 47.5)
  arc A11 (45.75, 47.5) -> (44, 49.25) centre (44, 47.5) ccw
  line L12 (44, 49.25) -> (-44, 49.25)
  arc A12 (-44, 49.25) -> (-45.75, 47.5) centre (-44, 47.5) ccw
  line L13 (-45.75, -49.25) -> (0, -49.25) construction
  line L14 (0, -49.25) -> (0, -29.25) construction
  line L15 (0, -29.25) -> (-45.75, -29.25) construction
  line L16 (-45.75, -29.25) -> (-45.75, -49.25) construction
  circle A13 centre (0, -30) radius 5
  circle A14 centre (0, -30) radius 4
  circle A15 centre (0, -30) radius 3
  circle A16 centre (0, -30) radius 2
  circle A17 centre (0, -30) radius 1
  line L17 (5, -28.5) -> (-5, -28.5)
  line L18 (-5, -28.5) -> (-5, -31.5)
  line L19 (-5, -31.5) -> (5, -31.5)
  line L20 (5, -31.5) -> (5, -28.5)
  line L21 (5, -28.5) -> (-5, -31.5) construction
  line L22 (-5, -28.5) -> (5, -31.5) construction
  line L23 (1.5, -35.5) -> (-1.5, -35.5)
  line L24 (-1.5, -35.5) -> (-1.5, -24.5)
  line L25 (-1.5, -24.5) -> (1.5, -24.5)
  line L26 (1.5, -24.5) -> (1.5, -35.5)
  line L27 (1.5, -35.5) -> (-1.5, -24.5) construction
  line L28 (-1.5, -35.5) -> (1.5, -24.5) construction
  point P0 (0, -30)
  point P1 (0, -30)
  dimension "d420" = 20
  dimension "d421" = 10
  dimension "d422" = 8
  dimension "d423" = 6
  dimension "d424" = 4
  dimension "d425" = 2
  dimension "d426" = 10
  dimension "d427" = 3
  dimension "d428" = 3
  dimension "d429" = 11
  constraint horizontal L13
  constraint vertical L14
  constraint horizontal L15
  constraint vertical L16
  constraint coincident L14 P1
  constraint concentric A13 A14
  constraint concentric A13 A15
  constraint concentric A15 A16
  constraint concentric A15 A17
  constraint horizontal L17
  constraint perpendicular L17 L18
  constraint parallel L17 L19
  constraint parallel L18 L20
  constraint coincident L21 P1
  constraint coincident L22 P1
  constraint coincident P1 P0
  constraint horizontal L23
  constraint perpendicular L23 L24
  constraint parallel L23 L25
  constraint parallel L24 L26
  constraint coincident L27 P1
  constraint coincident L28 P1
  measures "d420" distance of L13.start L15.end
  measures "d421" diameter of A13
  measures "d422" diameter of A14
  measures "d423" diameter of A15
  measures "d424" diameter of A16
  measures "d425" diameter of A17
  measures "d426" distance of L18.end L19.end
  measures "d427" distance of L17.end L18.end
  measures "d428" distance of L24.end L25.end
  measures "d429" distance of L23.end L24.end
extrude "Extrude4''" cut sketch "Sketch4 (3)" against normal blind 1.75 contours A13 A14 L17 L26 | A13 A14 L19 L26 | A13 A14 L24 L26 | A13 A14 L24 L26 | A13 A14 L17 L24 | A15 L17 L26 | A15 A16 L17 L19 L26 | A13 A14 L19 L24 | A15 L19 L26 | A15 L17 L24 | A15 L19 L24 | A15 A16 L17 L19 L24 bodies 3 in component "Smart_Chair_Board_Case_Top_Cover"
sketch "Sketch5 (3)" plane through (0, 36.75, 0) normal (0, 1, 0) x (-1, 0, 0) in component "Smart_Chair_Board_Case_Top_Cover"
  arc A0 (-4.7697, -31.5) -> (4.7697, -31.5) centre (0, -30) ccw
  line L0 (-4.7697, -31.5) -> (-3.7081, -31.5)
  arc A1 (-3.7081, -31.5) -> (3.7081, -31.5) centre (0, -30) ccw
  line L1 (3.7081, -31.5) -> (4.7697, -31.5)
  arc A2 (1.5, -32.5981) -> (1.5, -27.4019) centre (0, -30) ccw
  line L2 (1.5, -32.5981) -> (1.5, -31.3229)
  arc A3 (1.5, -31.3229) -> (1.5, -28.6771) centre (0, -30) ccw
  line L3 (1.5, -28.6771) -> (1.5, -27.4019)
  arc A4 (4.7697, -28.5) -> (-4.7697, -28.5) centre (0, -30) ccw
  line L4 (4.7697, -28.5) -> (3.7081, -28.5)
  arc A5 (3.7081, -28.5) -> (-3.7081, -28.5) centre (0, -30) ccw
  line L5 (-3.7081, -28.5) -> (-4.7697, -28.5)
  arc A6 (-1.5, -27.4019) -> (-1.5, -32.5981) centre (0, -30) ccw
  line L6 (-1.5, -27.4019) -> (-1.5, -28.6771)
  arc A7 (-1.5, -28.6771) -> (-1.5, -31.3229) centre (0, -30) ccw
  line L7 (-1.5, -31.3229) -> (-1.5, -32.5981)
  circle A8 centre (30.25, 0.75) radius 2.8
  circle A9 centre (30.25, -10.25) radius 2.8
  circle A10 centre (30.25, -21.25) radius 2.8
  circle A11 centre (-49.25, 0) radius 1
  circle A12 centre (0, -52.75) radius 1
  circle A13 centre (49.25, 0) radius 1
  line L8 (-45.75, 47.5) -> (-45.75, 3.5)
  line L9 (-45.75, 3.5) -> (-49.25, 3.5)
  arc A14 (-49.25, 3.5) -> (-49.25, -3.5) centre (-49.25, 0) ccw
  line L10 (-49.25, -3.5) -> (-45.75, -3.5)
  line L11 (-45.75, -3.5) -> (-45.75, -47.5)
  arc A15 (-45.75, -47.5) -> (-44, -49.25) centre (-44, -47.5) ccw
  line L12 (-44, -49.25) -> (-3.5, -49.25)
  line L13 (-3.5, -49.25) -> (-3.5, -52.75)
  arc A16 (-3.5, -52.75) -> (3.5, -52.75) centre (0, -52.75) ccw
  line L14 (3.5, -52.75) -> (3.5, -49.25)
  line L15 (3.5, -49.25) -> (44, -49.25)
  arc A17 (44, -49.25) -> (45.75, -47.5) centre (44, -47.5) ccw
  line L16 (45.75, -47.5) -> (45.75, -3.5)
  line L17 (45.75, -3.5) -> (49.25, -3.5)
  arc A18 (49.25, -3.5) -> (49.25, 3.5) centre (49.25, 0) ccw
  line L18 (49.25, 3.5) -> (45.75, 3.5)
  line L19 (45.75, 3.5) -> (45.75, 47.5)
  arc A19 (45.75, 47.5) -> (44, 49.25) centre (44, 47.5) ccw
  line L20 (44, 49.25) -> (-44, 49.25)
  arc A20 (-44, 49.25) -> (-45.75, 47.5) centre (-44, 47.5) ccw
  line L21 (30.25, -21.25) -> (-31.25, -21.25) construction
  line L22 (30.25, 0.75) -> (-31.25, 0.75) construction
  circle A21 centre (-31.25, -21.25) radius 6.5
  circle A22 centre (-31.25, 0.75) radius 6.5
  dimension "d432" = 61.5
  dimension "d433" = 61.5
  dimension "d434" = 13
  dimension "d435" = 13
  constraint coincident A10.centre L21.start
  constraint perpendicular L11 L21
  constraint coincident A8.centre L22.start
  constraint horizontal L22
  constraint coincident L21.end A21.centre
  constraint coincident L22.end A22.centre
  measures "d432" distance of A10.centre L21.end
  measures "d433" distance of A8.centre L22.end
  measures "d434" diameter of A21
  measures "d435" diameter of A22
extrude "Extrude5''" cut sketch "Sketch5 (3)" against normal blind 1.75 contours A21 | A22 bodies 3 in component "Smart_Chair_Board_Case_Top_Cover"
sketch "Sketch1 (5)" plane through (0, 43, 0) normal (0, 1, 0) x (-1, 0, 0) in component "Smart_Sprayer_Board_Case_Cover"
  line L0 (-76.75, 47.5) -> (76.75, 47.5)
  arc A0 (77.5, 46.75) -> (76.75, 47.5) centre (76.75, 46.75) ccw
  line L1 (77.5, 46.75) -> (77.5, -46.75)
  arc A1 (76.75, -47.5) -> (77.5, -46.75) centre (76.75, -46.75) ccw
  line L2 (76.75, -47.5) -> (-76.75, -47.5)
  arc A2 (-77.5, -46.75) -> (-76.75, -47.5) centre (-76.75, -46.75) ccw
  line L3 (-77.5, -46.75) -> (-77.5, 46.75)
  arc A3 (-76.75, 47.5) -> (-77.5, 46.75) centre (-76.75, 46.75) ccw
  arc A4 (79.25, 47.5) -> (77.5, 49.25) centre (77.5, 47.5) ccw
  line L4 (77.5, 49.25) -> (-77.5, 49.25)
  arc A5 (-77.5, 49.25) -> (-79.25, 47.5) centre (-77.5, 47.5) ccw
  line L5 (-79.25, 47.5) -> (-79.25, -47.5)
  arc A6 (-79.25, -47.5) -> (-77.5, -49.25) centre (-77.5, -47.5) ccw
  line L6 (-77.5, -49.25) -> (77.5, -49.25)
  arc A7 (77.5, -49.25) -> (79.25, -47.5) centre (77.5, -47.5) ccw
  line L7 (79.25, -47.5) -> (79.25, 47.5)
extrude "Extrude1'''" add sketch "Sketch1 (5)" against normal blind 5 separate body contours L0 A0 L1 A1 L2 A2 L3 A3 makes body 4 in component "Smart_Sprayer_Board_Case_Cover"
shell "Shell1" thickness 1.5 removed faces 1 at (-25.5833, 43, -15.8333) on bodies 4 in component "Smart_Sprayer_Board_Case_Cover"
extrude "Extrude2'''" cut 1 faces at (25.3333, 39.5, -15.3333) along direction (0, -1, 0) blind 1.5 on bodies 4 bodies 4 in component "Smart_Sprayer_Board_Case_Cover"
sketch "Sketch2 (4)" plane through (0, 43, 0) normal (0, 1, 0) x (-1, 0, 0) in component "Smart_Sprayer_Board_Case_Cover"
  line L0 (-76.75, 47.5) -> (76.75, 47.5)
  arc A0 (77.5, 46.75) -> (76.75, 47.5) centre (76.75, 46.75) ccw
  line L1 (77.5, 46.75) -> (77.5, -46.75)
  arc A1 (76.75, -47.5) -> (77.5, -46.75) centre (76.75, -46.75) ccw
  line L2 (76.75, -47.5) -> (-76.75, -47.5)
  arc A2 (-77.5, -46.75) -> (-76.75, -47.5) centre (-76.75, -46.75) ccw
  line L3 (-77.5, -46.75) -> (-77.5, 46.75)
  arc A3 (-76.75, 47.5) -> (-77.5, 46.75) centre (-76.75, 46.75) ccw
  arc A4 (79.25, 47.5) -> (77.5, 49.25) centre (77.5, 47.5) ccw
  line L4 (77.5, 49.25) -> (-77.5, 49.25)
  arc A5 (-77.5, 49.25) -> (-79.25, 47.5) centre (-77.5, 47.5) ccw
  line L5 (-79.25, 47.5) -> (-79.25, -47.5)
  arc A6 (-79.25, -47.5) -> (-77.5, -49.25) centre (-77.5, -47.5) ccw
  line L6 (-77.5, -49.25) -> (77.5, -49.25)
  arc A7 (77.5, -49.25) -> (79.25, -47.5) centre (77.5, -47.5) ccw
  line L7 (79.25, -47.5) -> (79.25, 47.5)
extrude "Extrude3'''" add sketch "Sketch2 (4)" along normal blind 1.75 contours L0 A0 L1 A1 L2 A2 L3 A3 | A4 L4 A5 L5 A6 L6 A7 L7 bodies 4 in component "Smart_Sprayer_Board_Case_Cover"
extrude "Extrude4'''" cut 1 faces at (25.3333, 41.3333, 46) along direction (0, 0, 1) blind 0.2 on bodies 4 bodies 4 in component "Smart_Sprayer_Board_Case_Cover"
extrude "Extrude5'''" cut 1 faces at (76, 39.6667, -15.2667) along direction (1, 0, 0) blind 0.2 on bodies 4 bodies 4 in component "Smart_Sprayer_Board_Case_Cover"
extrude "Extrude6''" cut 1 faces at (-76, 41.3333, 15.4667) along direction (-1, 0, 0) blind 0.2 on bodies 4 bodies 4 in component "Smart_Sprayer_Board_Case_Cover"
extrude "Extrude7''" cut 1 faces at (-25.4, 39.6667, -46) along direction (0, 0, -1) blind 0.2 on bodies 4 bodies 4 in component "Smart_Sprayer_Board_Case_Cover"
component "Smart_Sprayer_Board_Case" placed x (1, 0, 0) y (0, 1, 0) z (0, 0, 1) at (0, 0, 0)
component "Smart_Chair_Board_Case_Top" placed x (1, 0, 0) y (0, 1, 0) z (0, 0, 1) at (0, 0, 0)
component "Smart_Chair_Board_Case_Top_Cover" placed x (1, 0, 0) y (0, 1, 0) z (0, 0, 1) at (0, 0, 0)
component "Smart_Sprayer_Board_Case_Cover" placed x (1, 0, 0) y (0, 1, 0) z (0, 0, 1) at (0, 0, 0)
equation "ScrewholeDia = 2 mm"
equation "ShaftOuterDia = 4.8 mm"
equation "ShaftSplinesInnerDia = 4.5 mm"
equation "NumSplines = 20"
equation "SplineTipPointiness = ShaftOuterDia * PI / NumSplines / 8"
equation "SplineInnerPointiness = ShaftOuterDia * PI / NumSplines / 8"
equation "ShaftHeight = 3.5 mm"
equation "ShaftScrewSectionsize = 0.2 mm"
equation "ShaftScrewPitch = ShaftHeight / 0.4 mm"
equation "HatDia = 11.5 mm"
equation "n = 14.5 mm"
equation "HatTipDia = 5.5 mm"
equation "HatHeight = 4.5 mm"
equation "Hole_to_closest_end_dist = HatDia / 2"
equation "ServoBodyLength = 22.4 mm"
equation "ServoBodyWidth = 12.4 mm"
equation "ServoBodyHeight = 24 mm"
equation "ServoCornerWireRecess = 3 mm"
equation "ServoTabRecess = -4.4 mm"
equation "ServoTabSize = 5 mm"
equation "ServoHoleRecess = 3.6 mm"
equation "TabScrewSize = 2.6 mm"
equation "TabScrewGapSize = 1.2 mm"
equation "TabThickness = -2.4 mm"
equation "WireHoleWidth = 3 mm"
equation "WireHoleOffset = 0.4 mm"
equation "WireHoleHeight = 2 mm"
equation "WireLenght = 5 mm"
equation "OuterHubDia = 7.3 mm + 2 * tol"
equation "InnerHubDia = 4.65 mm"
equation "MajorArmLen = 36.2 mm + 2 * tol"
equation "MinroArmLen = 19 mm + 2 * tol"
equation "TipDiaMajor = 5 mm + 2 * tol"
equation "TipDiaMinor = 4 mm + 2 * tol"
equation "ScrewHole = 2.5 mm"
equation "DriveHole = 2 mm"
equation "d14 = DriveHole"
equation "d19 = OuterHubDia + 1.5 mm + tol + 2 * tol"
equation "ReinforcerWidth = 1 mm + 2 * tol"
equation "HoleSlideAdj = 0.6 mm"
equation "SideHoleSlideAdj = 0.25 mm"
equation "HornCollarDepth = -2.7 mm"
equation "HornUnderside = -1 mm"
equation "HornInnerScrewTabThickness = 1.2 mm"
equation "HornUpperHeight = 2.3 mm"
equation "HornArmTopSide = -1.5 mm"
equation "TrayGap = 0.2 mm"
equation "TraySideWidth = 3 mm"
equation "TrayEndExtraMinus1 = 1 mm - TrayGap"
equation "ServoTrayThickness = 3 mm"
